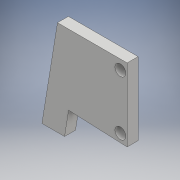
# Autodesk Inventor part: garra
Saved by Autodesk Inventor 2018 (Build 220112000, 112)
## iProperties
Created: 2018-05-25
Part Number: garra
Material: Generic
Document SubType Name: Modeling
Designer: vigus
Density: 1 g/cm^3
Appearance: Default
Author: vigus
Autodesk Inventor part; units mm, degrees
ref_plane "YZ Plane" through (0, 0, 0) normal (1, 0, 0) x (0, 1, 0)
ref_plane "XZ Plane" through (0, 0, 0) normal (0, 1, 0) x (-1, 0, 0)
ref_plane "XY Plane" through (0, 0, 0) normal (0, 0, 1) x (1, 0, 0)
sketch "Sketch1" plane through (0, 0, 0) normal (0, 1, 0) x (-1, 0, 0)
  line L0 (0, -4.2684) -> (0, 15.7316)
  line L1 (0, 15.7316) -> (19.1343, 15.7316)
  line L2 (19.1343, 15.7316) -> (23.407, -10.3664)
  line L3 (23.407, -10.3664) -> (17.192, -10.3664)
  line L4 (17.192, -10.3664) -> (16.0766, -3.5534)
  line L5 (16.0766, -3.5534) -> (0, -4.2684)
  circle A0 centre (1.8613, 13.0905) radius 1.5
  circle A1 centre (1.8613, -1.9095) radius 1.5
  point P0 (0, 0)
  dimension "d0" = 3
  dimension "d1" = 3
  dimension "d2" = 15
  dimension "d3" = 20
  constraints: 12 end point, 2 centre point, 2 parallel, 1 perpendicular, 1 vertical
  measures "d0" diameter of A0
  measures "d1" diameter of A1
  measures "d2" distance of A1.centre A0.centre
  measures "d3" distance of L0.start L0.end
extrude "Extrusion1" add sketch "Sketch1" along normal blind 3
body "Solid1"
